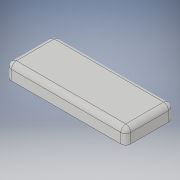
# Autodesk Inventor part: box_top
Saved by Autodesk Inventor 2017 (Build 210142000, 142)
## iProperties
Created: 2017-09-23
Part Number: box_top
Material: Generic
Document SubType Name: Modeling
Designer: Mitch
Density: 1 g/cm^3
Appearance: Default
Author: Mitch
Autodesk Inventor part; units mm, degrees
ref_plane "YZ Plane" through (0, 0, 0) normal (1, 0, 0) x (0, 1, 0)
ref_plane "XZ Plane" through (0, 0, 0) normal (0, 1, 0) x (-1, 0, 0)
ref_plane "XY Plane" through (0, 0, 0) normal (0, 0, 1) x (1, 0, 0)
sketch "Sketch1" plane through (0, 0, 0) normal (0, 1, 0) x (-1, 0, 0)
  line L0 (0, 0) -> (76.2, 0)
  line L1 (76.2, 0) -> (76.2, -30.48)
  line L2 (76.2, -30.48) -> (0, -30.48)
  line L3 (0, -30.48) -> (0, 0)
  dimension "d0" = 76.2
  dimension "d1" = 30.48
  constraints: 8 end point, 2 parallel, 1 horizontal, 1 perpendicular
  measures "d0" distance of L1.end L2.end
  measures "d1" distance of L0.end L1.end
extrude "Extrusion1" add sketch "Sketch1" along normal blind 9.525
fillet "Fillet1" radius 3.175 8 edges at (0, 4.7625, 0) (0, 9.525, -15.24) (-38.1, 9.525, 0) (-38.1, 9.525, -30.48) (0, 4.7625, -30.48) (-76.2, 4.7625, 0) (-76.2, 9.525, -15.24) (-76.2, 4.7625, -30.48)
shell "Shell1" thickness 2.54 removed faces 1 at (-26.4583, 0, -20.32)
sketch "Sketch2" plane through (0, 0, 0) normal (0, -1, 0) x (1, 0, 0)
  line L0 (0, -27.305) -> (0, -3.175) projected
  arc A0 (-3.175, -30.48) -> (0, -27.305) centre (-3.175, -27.305) ccw projected
  line L1 (-73.025, -30.48) -> (-3.175, -30.48) projected
  arc A1 (0, -3.175) -> (-3.175, 0) centre (-3.175, -3.175) ccw projected
  line L2 (-3.175, 0) -> (-73.025, 0) projected
  arc A2 (-73.025, 0) -> (-76.2, -3.175) centre (-73.025, -3.175) ccw projected
  line L3 (-76.2, -3.175) -> (-76.2, -27.305) projected
  arc A3 (-76.2, -27.305) -> (-73.025, -30.48) centre (-73.025, -27.305) ccw projected
  arc A4 (-73.025, -1.27) -> (-74.93, -3.175) centre (-73.025, -3.175) ccw
  line L4 (-73.025, -1.27) -> (-3.175, -1.27)
  arc A5 (-1.27, -3.175) -> (-3.175, -1.27) centre (-3.175, -3.175) ccw
  line L5 (-1.27, -3.175) -> (-1.27, -27.305)
  arc A6 (-3.175, -29.21) -> (-1.27, -27.305) centre (-3.175, -27.305) ccw
  line L6 (-3.175, -29.21) -> (-73.025, -29.21)
  arc A7 (-74.93, -27.305) -> (-73.025, -29.21) centre (-73.025, -27.305) ccw
  line L7 (-74.93, -27.305) -> (-74.93, -3.175)
  point P0 (0, 0)
  dimension "d6" = 1.27
  constraints: 8 end point, 8 point on circle, 4 centre point, 7 other
  measures "d6" radial gap between concentric circles of A2 A4
extrude "Extrusion2" cut sketch "Sketch2" against normal blind 1.27 contours L4 A5 L5 A6 L6 A7 L7 A4
body "Solid1"
